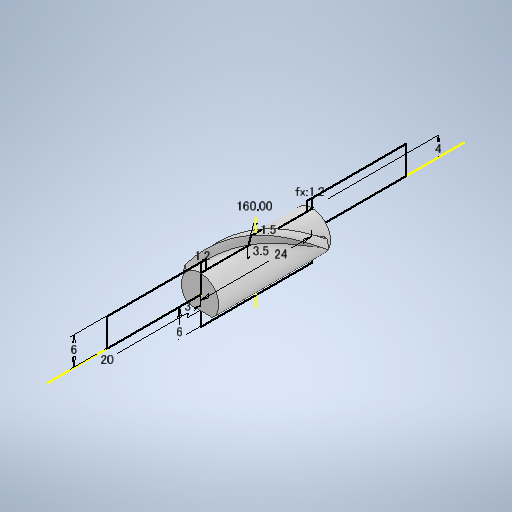
# Autodesk Inventor part: SwitchLeverUnit_Roller
Saved by Autodesk Inventor 2025.1 (Build 291241000, 241)
## iProperties
Created: 2025-03-08
Part Number: SwitchLeverUnit_Roller
Material: 一般
Document SubType Name: Modeling
Designer: kumagai
Density: 1 g/cm^3
Appearance: 既定
Author: kumagai
Autodesk Inventor part; units mm, degrees
ref_plane "YZ Plane" through (0, 0, 0) normal (1, 0, 0) x (0, 1, 0)
ref_plane "XZ Plane" through (0, 0, 0) normal (0, 1, 0) x (-1, 0, 0)
ref_plane "XY Plane" through (0, 0, 0) normal (0, 0, 1) x (1, 0, 0)
sketch "ProfileSketch" plane through (0, 0, 0) normal (1, 0, 0) x (0, 1, 0)
  line L0 (0, 44.8) -> (0, -44.8) projected
  line L1 (-8.4, 0) -> (8.4, 0) projected
  line L2 (0, 12) -> (4, 12)
  line L3 (4, 12) -> (4, -12)
  line L4 (4, -12) -> (0, -12)
  line L5 (0, 12) -> (6, 12)
  line L6 (6, 12) -> (6, 32)
  line L7 (6, 32) -> (0, 32)
  line L8 (0, 32) -> (0, 12)
  line L9 (0, -12) -> (6, -12)
  line L10 (6, -12) -> (6, -32)
  line L11 (6, -32) -> (0, -32)
  line L12 (0, -32) -> (0, -12)
  line L13 (4, 1.75) -> (5.5, 1.204)
  line L14 (5.5, 1.204) -> (5.5, -1.204)
  line L15 (5.5, -1.204) -> (4, -1.75)
  line L16 (4, 10.8) -> (6, 10.8)
  line L17 (6, 10.8) -> (6, 12)
  line L18 (6, -12) -> (6, -10.8)
  line L19 (6, -10.8) -> (4, -10.8)
  line L20 (-3, 12) -> (-6, 12)
  line L21 (-6, 12) -> (-6, -12)
  line L22 (-6, -12) -> (-3, -12)
  line L23 (-3, -12) -> (-3, 12)
  point P0 (0, 0)
  point P1 (0, -31)
  point P2 (0, 32)
  dimension "d0" = 24
  dimension "d1" = 4
  dimension "d2" = 20
  dimension "d3" = 6
  dimension "d4" = 3.5
  dimension "d5" = 20
  dimension "d6" = 1.5
  dimension "d25" = 1.2
  dimension "d26" = 1.2
  dimension "d27" = 3
  dimension "d28" = 6
  constraints: 44 end point, 7 point on line, 4 collinear, 4 symmetric about line, 1 horizontal, 1 vertical, 2 other
  measures "d0" distance between parallel lines of L4 L2
  measures "d1" distance between parallel lines of L0 L3
  measures "d2" distance between parallel lines of L7 L5
  measures "d3" distance between parallel lines of L8 L6
  measures "d4" distance of L15.end L13.start
  measures "d5" angle of L1 L13
  measures "d6" distance between parallel lines of L3 L14
  measures "d25" distance between parallel lines of L5 L16
  measures "d26" distance between parallel lines of L19 L9
  measures "d27" distance between parallel lines of L23 L0
  measures "d28" distance between parallel lines of L0 L21
revolve "RollerBody" add sketch "ProfileSketch" angle 360 about axis through (0, 0, 0) along (0, 0, -1) contours L2 L3 L1 L0 | L1 L3 L4 L0
coil "Screw1" sketch "ProfileSketch" operation add axis through (0, 0, 0) along (0, 0, -1) pitch 45 turns 0.466667 hand right contours L3 L13 L14 L1 | L1 L14 L15 L3
coil "Screw2" sketch "ProfileSketch" operation add axis through (0, 0, 0) along (0, 0, 1) pitch 45 turns 0.466667 hand right contours L3 L13 L14 L1 | L1 L14 L15 L3
revolve "Cutoff1" cut sketch "ProfileSketch" angle 360 about axis through (0, 0, 0) along (0, 0, -1) contours L7 L6 L5 L2 L0 | L5 L17 L16 L3 | L4 L9 L10 L11 L0 | L3 L19 L18 L9
extrude "FlatFace" cut sketch "ProfileSketch" along normal through all both and the other way through all contours L21 L20 L23 L1 | L1 L23 L22 L21
sketch "スケッチ2" plane through (-2.6458, -3, 12) normal (0, -1, 0) x (1, 0, 0)
  line L0 (0, -24) -> (0, 0) projected
  line L1 (5.2915, 0) -> (5.2915, -24) projected
  line L2 (2.6458, 4.8) -> (2.6458, -28.8) projected
  line L3 (-5.0542, -12) -> (10.3458, -12) projected
  line L4 (3.6958, -5) -> (1.5958, -5)
  line L5 (1.5958, -5) -> (1.5958, -19)
  line L6 (1.5958, -19) -> (3.6958, -19)
  line L7 (3.6958, -19) -> (3.6958, -5)
  point P0 (2.6458, -12)
  dimension "d32" = 2.1
  dimension "d33" = 14
  constraints: 8 end point, 2 other
  measures "d32" distance between parallel lines of L5 L7
  measures "d33" distance between parallel lines of L6 L4
extrude "LeverSlot" cut sketch "スケッチ2" against normal blind 4
chamfer "LeverSlotChamfer" distance 4 angle 45 2 edges at (0, 1, 7) (0, 1, -7)
chamfer "ScrewEdge1" distance 0.75 distance2 1.5 1 edges at (-5.4891, 0.3453, 10.8) measured on face at (-5.4891, 0.3453, 10.3)
chamfer "ScrewEdge2" distance 0.75 distance2 1.5 1 edges at (5.4891, 0.3453, -10.8) measured on face at (5.4891, 0.3453, -10.3)
equation "\"d26\" = d25"
